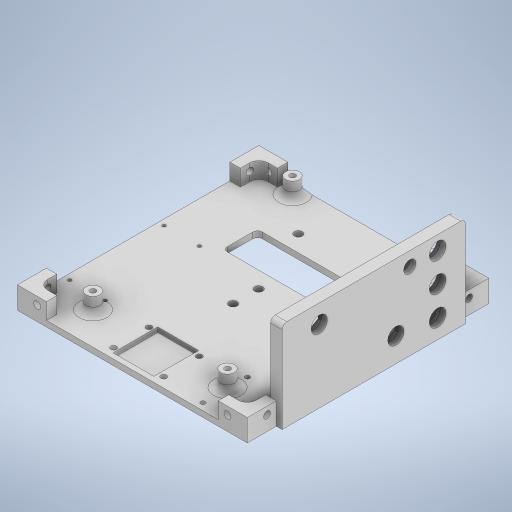
# Autodesk Inventor part: TA07 ELECTRONICS MOUNT REV 3
Saved by Autodesk Inventor 2024 (Build 280153000, 153)
## iProperties
Created: 2023-06-26
Part Number: TA07 ELECTRONICS MOUNT REV 3
Material: Generic
Document SubType Name: Modeling
Designer: TEST BENCH
Density: 1 g/cm^3
Appearance: Default
Author: TEST BENCH
Autodesk Inventor part; units mm, degrees
note: some values were not read from the file. Chosen so that the rebuilt part matches the saved one: direction of "Hole6"; direction of "Hole7".
ref_plane "YZ Plane" through (0, 0, 0) normal (1, 0, 0) x (0, 1, 0)
sketch "Sketch1" plane through (0, 0, 0) normal (0, 1, 0) x (-1, 0, 0)
  line L0 (0, 0) -> (99, 0)
  line L1 (99, 0) -> (99, -104)
  line L2 (99, -104) -> (0, -104)
  line L3 (0, -104) -> (0, 0)
  line L4 (61.8, -4.22) -> (40.2, -4.22) construction
  line L5 (40.2, -4.22) -> (40.2, -19.47) construction
  line L6 (40.2, -19.47) -> (61.8, -19.47) construction
  line L7 (61.8, -19.47) -> (61.8, -4.22) construction
  line L8 (52.5, -46.37) -> (52.5, -57.37) construction
  line L9 (64.5, -86.5) -> (37.5, -86.5) construction
  line L10 (65.8, 0) -> (36.2, 0)
  line L11 (36.2, 0) -> (36.2, -0.22)
  line L12 (36.2, -0.22) -> (65.8, -0.22)
  line L13 (65.8, -0.22) -> (65.8, 0)
  point P0 (51, -4.22)
  point P1 (36.2, 0)
  dimension "d0" = 104
  dimension "d1" = 99
  dimension "d2" = 11
  dimension "d3" = 27
  dimension "d5" = 15.25
  dimension "d6" = 21.6
  dimension "d8" = 26.9
  dimension "d11" = 17.5
  dimension "d12" = 4
  dimension "d13" = 4
  dimension "d14" = 4
  dimension "d147" = 29.13
  dimension "d202" = 2.7
  dimension "d203" = 61.5
  dimension "d204" = 46.5
  constraints: 28 end point, 8 parallel, 4 coincident, 3 horizontal, 3 perpendicular, 1 midpoint, 1 point on line
  measures "d0" distance of L0.end L1.end
  measures "d1" distance of L1.end L2.end
  measures "d2" distance of L8.end L8.start
  measures "d3" distance of L9.end L9.start
  measures "d5" distance of L6.end L4.start
  measures "d6" distance of L4.start L4.end
  measures "d8" vertical distance of L8.start L6.end
  measures "d11" distance from line of L2 L9.start
  measures "d12" distance between parallel lines of L13 L7
  measures "d13" distance from line of L12 point (51, -4.22)
  measures "d14" distance between parallel lines of L5 L11
  measures "d147" vertical distance of L9.end L8.end
  measures "d202" horizontal distance of L5.end L9.end
  measures "d203" horizontal distance of L1.end L9.end
  measures "d204" distance from line of L1 L8.end
extrude "Extrusion1" add sketch "Sketch1" against normal blind 2.5
hole "Hole1" at (-61.8, 0, -19.47) at (-61.8, 0, -4.22) at (-40.2, 0, -4.22) at (-40.2, 0, -19.47) direction (0, -1, 0) diameter 2.5 end through all
hole "Hole2" at (-52.5, 0, -46.37) at (-52.5, 0, -57.37) at (-64.5, 0, -86.5) at (-37.5, 0, -86.5) direction (0, -1, 0) diameter 3.5 end through all
sketch "Sketch2" plane through (0, -2.5, 0) normal (0, -1, 0) x (1, 0, 0)
  line L0 (-81.26, -20) -> (-96.5, -20) construction
  line L1 (-96.5, -20) -> (-96.5, -60.64) construction
  line L2 (-96.5, -60.64) -> (-81.26, -60.64) construction
  line L3 (-81.26, -60.64) -> (-81.26, -20) construction
  line L4 (-3, -36) -> (-22, -36) construction
  line L5 (-22, -36) -> (-22, -92) construction
  line L6 (-22, -92) -> (-3, -92) construction
  line L7 (-3, -92) -> (-3, -36) construction
  line L8 (-22.035, -3) -> (-22.035, -22.05) construction
  line L9 (0, -104) -> (0, 0) construction
  line L10 (-99, -104) -> (0, -104) projected
  line L11 (-12.035, -6) -> (-24.035, -6)
  line L12 (-24.035, -6) -> (-24.035, -19.05)
  line L13 (-24.035, -19.05) -> (-12.035, -19.05)
  line L14 (-12.035, -19.05) -> (-12.035, -6)
  line L15 (-0.525, -0.525) -> (-8.525, -0.525)
  line L16 (-8.525, -0.525) -> (-8.525, -24.525)
  line L17 (-8.525, -24.525) -> (-0.525, -24.525)
  line L18 (-0.525, -24.525) -> (-0.525, -0.525)
  line L19 (-0.9653, -37.5) -> (-7.5262, -37.5)
  line L20 (-7.5262, -37.5) -> (-7.5262, -51.2095)
  line L21 (-7.5262, -51.2095) -> (-0.9653, -51.2095)
  line L22 (-0.9653, -51.2095) -> (-0.9653, -37.5)
  line L23 (-13.4891, -37.5) -> (-25, -37.5)
  line L24 (-25, -37.5) -> (-25, -90.5)
  line L25 (-25, -90.5) -> (-13.4891, -90.5)
  line L26 (-13.4891, -90.5) -> (-13.4891, -37.5)
  line L27 (-79.76, -21.5) -> (-98, -21.5)
  line L28 (-98, -21.5) -> (-98, -59.14)
  line L29 (-98, -59.14) -> (-79.76, -59.14)
  line L30 (-79.76, -59.14) -> (-79.76, -21.5)
  circle A0 centre (-52.5, -57.37) radius 1.75 construction
  circle A1 centre (-64.5, -86.5) radius 1.75 construction
  line L31 (-25, -64.435) -> (-75, -64.435)
  line L32 (-75, -64.435) -> (-75, -79.435)
  line L33 (-75, -79.435) -> (-25, -79.435)
  line L34 (-25, -79.435) -> (-25, -64.435)
  line L35 (-99, 0) -> (-99, -104) projected
  line L36 (-82.7648, -21.5) -> (-94.7648, -21.5)
  line L37 (-94.7648, -21.5) -> (-94.7648, -6)
  line L38 (-94.7648, -6) -> (-82.7648, -6)
  line L39 (-82.7648, -6) -> (-82.7648, -21.5)
  line L40 (-2.5, -28.2417) -> (-10.5305, -28.2417)
  line L41 (-10.5305, -28.2417) -> (-10.5305, -31.9874)
  line L42 (-10.5305, -31.9874) -> (-2.5, -31.9874)
  line L43 (-2.5, -31.9874) -> (-2.5, -28.2417)
  line L44 (-0.191, -24.844) -> (-24.829, -24.844) construction
  line L45 (-24.829, -24.844) -> (-24.829, -0.206) construction
  line L46 (-24.829, -0.206) -> (-0.191, -0.206) construction
  line L47 (-0.191, -0.206) -> (-0.191, -24.844) construction
  line L48 (0, 0) -> (-99, 0) construction
  point P0 (-96.5, -60.64)
  point P1 (-24.035, -12.525)
  point P2 (-4.525, -24.525)
  point P3 (-4.525, -0.525)
  point P4 (-19.2445, -90.5)
  point P5 (-88.88, -20)
  point P6 (-8.525, -12.525)
  point P7 (-0.525, -12.525)
  point P8 (-25, -79.435)
  point P9 (-88.88, -21.5)
  point P10 (-75, -71.935)
  point P11 (-2.5, -30.1145)
  dimension "d32" = 19.05
  dimension "d33" = 19
  dimension "d34" = 56
  dimension "d35" = 3
  dimension "d36" = 12
  dimension "d39" = 40.64
  dimension "d40" = 15.24
  dimension "d42" = 3
  dimension "d43" = 3
  dimension "d44" = 12
  dimension "d46" = 24
  dimension "d47" = 2.475
  dimension "d48" = 1.5
  dimension "d49" = 1.5
  dimension "d50" = 1.5
  dimension "d51" = 1.5
  dimension "d52" = 1.5
  dimension "d53" = 1.5
  dimension "d56" = 15
  dimension "d58" = 50
  dimension "d59" = 8
  dimension "d148" = 1
  dimension "d189" = 29.13
  dimension "d190" = 14.565
  dimension "d191" = 25
  dimension "d192" = 12
  dimension "d193" = 15.5
  dimension "d196" = 2.5
  dimension "d221" = 24.638
  dimension "d222" = 24.638
  dimension "d223" = 2.794
  dimension "d224" = 3
  dimension "d226" = 0.334
  dimension "d227" = 0.794
  dimension "d229" = 2.794
  dimension "d230" = 0.525
  dimension "d231" = 0.525
  constraints: 90 end point, 22 parallel, 11 horizontal, 11 perpendicular, 10 coincident, 10 midpoint, 2 point on line, 1 collinear, 1 vertical
  measures "d32" distance of L8.start L8.end
  measures "d33" distance of L5.end L6.end
  measures "d34" distance of L6.end L4.start
  measures "d35" distance between parallel lines of L9 L7
  measures "d36" distance between parallel lines of L10 L6
  measures "d39" distance of L2.end L0.start
  measures "d40" distance of L0.start L0.end
  measures "d42" distance from line of L8.start L11
  measures "d43" distance from line of L8.end L13
  measures "d44" distance from line of point (-24.035, -12.525) L14
  measures "d46" distance of point (-4.525, -24.525) point (-4.525, -0.525)
  measures "d47" distance from line of L15 point (-22.035, -3)
  measures "d48" distance from line of L4.end L23
  measures "d49" vertical distance of L5.end point (-19.245, -90.5)
  measures "d50" distance from line of L0.start L27
  measures "d51" distance from line of L2.end L29
  measures "d52" distance from line of point (-96.5, -60.64) L28
  measures "d53" distance between parallel lines of L3 L30
  measures "d56" distance between parallel lines of L33 L31
  measures "d58" distance between parallel lines of L32 L34
  measures "d59" distance of point (-8.525, -12.525) point (-0.525, -12.525)
  measures "d148" distance between parallel lines of L35 L28
  measures "d189" vertical distance of A0.centre A1.centre
  measures "d190" vertical distance of A1.centre point (-75, -71.935)
  measures "d191" distance between parallel lines of L9 L24
  measures "d192" distance between parallel lines of L37 L39
  measures "d193" distance between parallel lines of L27 L38
  measures "d196" distance from line of L9 point (-2.5, -30.115)
  measures "d221" distance of L46.end L44.start
  measures "d222" distance between parallel lines of L45 L47
  measures "d223" distance from line of L46 point (-22.035, -3)
  measures "d224" distance from line of L48 point (-22.035, -3)
  measures "d226" distance between parallel lines of L47 L18
  measures "d227" distance between parallel lines of L45 L12
  measures "d229" distance between parallel lines of L45 L8
  measures "d230" distance between parallel lines of L48 L15
  measures "d231" distance between parallel lines of L9 L18
extrude "Extrusion2" cut sketch "Sketch2" against normal through all
hole "Hole3" at (-81.26, -2.5, -20) at (-81.26, -2.5, -60.64) at (-96.5, -2.5, -60.64) at (-96.5, -2.5, -20) direction (0, 1, 0) diameter 1.5 end through all
hole "Hole4" at (-22.035, -2.5, -22.05) at (-22.035, -2.5, -3) direction (0, 1, 0) diameter 2 end through all
hole "Hole5" at (-3, -2.5, -36) at (-22, -2.5, -36) at (-3, -2.5, -92) at (-22, -2.5, -92) direction (0, 1, 0) diameter 2.5 end through all
sketch "Sketch3" plane through (0, 0, 0) normal (0, 1, 0) x (1, 0, 0)
  line L0 (-60.05, 2.22) -> (-42.45, 2.22)
  line L1 (-42.45, 2.22) -> (-42.45, 21.47)
  line L2 (-42.45, 21.47) -> (-60.05, 21.47)
  line L3 (-60.05, 21.47) -> (-60.05, 2.22)
  circle A0 centre (-61.8, 4.22) radius 1.25 projected
  circle A1 centre (-40.2, 4.22) radius 1.25 projected
  circle A2 centre (-40.2, 19.47) radius 1.25 projected
  point P0 (0, 0)
  dimension "d83" = 3
  dimension "d84" = 2
  dimension "d86" = 1
  dimension "d146" = 2
  constraints: 8 end point, 2 parallel, 1 horizontal, 1 perpendicular
  measures "d84" distance from line of A1.centre L0
  measures "d86" distance edge to line of A2 L1
  measures "d146" distance from line of A2.centre L2
extrude "Extrusion3" cut sketch "Sketch3" against normal through all contours L3 L2 L1 L0
sketch "Sketch4" plane through (0, 0, 0) normal (0, 1, 0) x (1, 0, 0)
  line L0 (-80.5, 14) -> (-22.5, 14) construction
  line L1 (-22.5, 14) -> (-22.5, 100) construction
  line L2 (-22.5, 100) -> (-80.5, 100) construction
  line L3 (-80.5, 100) -> (-80.5, 14) construction
  circle A0 centre (-80.5, 14) radius 3
  circle A1 centre (-80.5, 14) radius 1.25
  circle A2 centre (-80.5, 100) radius 3
  circle A3 centre (-80.5, 100) radius 1.25
  circle A4 centre (-22.5, 100) radius 3
  circle A5 centre (-22.5, 100) radius 1.25
  circle A6 centre (-22.5, 14) radius 3
  circle A7 centre (-22.5, 14) radius 1.25
  line L4 (-99, 0) -> (0, 0) projected
  line L5 (-99, 104) -> (-99, 0) projected
  line L6 (0, 104) -> (-99, 104) projected
  point P0 (-65.136, 0)
  point P1 (-64.63, 0)
  dimension "d90" = 18.5
  dimension "d91" = 86
  dimension "d92" = 58
  dimension "d93" = 2.5
  dimension "d94" = 2.5
  dimension "d95" = 2.5
  dimension "d96" = 2.5
  dimension "d97" = 6
  dimension "d98" = 6
  dimension "d99" = 6
  dimension "d100" = 6
  dimension "d167" = 4
  constraints: 8 centre point, 8 coincident, 8 end point, 2 parallel, 1 horizontal, 1 perpendicular
  measures "d90" distance from line of L5 L0.start
  measures "d91" distance of L2.end L0.start
  measures "d92" distance of L0.start L0.end
  measures "d93" diameter of A1
  measures "d94" diameter of A3
  measures "d95" diameter of A5
  measures "d96" diameter of A7
  measures "d97" diameter of A0
  measures "d98" diameter of A2
  measures "d99" diameter of A4
  measures "d100" diameter of A6
  measures "d167" distance from line of A2.centre L6
extrude "Extrusion4" add sketch "Sketch4" along normal blind 7
sketch "Sketch5" plane through (0, 0, 0) normal (0, 1, 0) x (1, 0, 0)
  line L0 (-99, 104) -> (-99, 0) projected
  line L1 (0, 0) -> (0, 104) projected
  line L2 (-99, 0) -> (0, 0)
  line L3 (0, 0) -> (0, 104)
  line L4 (0, 104) -> (-99, 104)
  line L5 (-99, 104) -> (-99, 0)
  circle A0 centre (-96.5, 20) radius 0.75 projected
  circle A1 centre (-81.26, 20) radius 0.75 projected
  circle A2 centre (-61.8, 19.47) radius 1.25 projected
  circle A3 centre (-40.2, 19.47) radius 1.25 projected
  circle A4 centre (-96.5, 60.64) radius 0.75 projected
  circle A5 centre (-81.26, 60.64) radius 0.75 projected
  circle A6 centre (-64.5, 86.5) radius 1.75 projected
  circle A7 centre (-52.5, 57.37) radius 1.75 projected
  circle A8 centre (-52.5, 46.37) radius 1.75 projected
  circle A9 centre (-22, 36) radius 1.25 projected
  circle A10 centre (-37.5, 86.5) radius 1.75 projected
  circle A11 centre (-3, 92) radius 1.25 projected
  circle A12 centre (-22, 92) radius 1.25 projected
  circle A13 centre (-3, 36) radius 1.25 projected
  circle A14 centre (-22.035, 22.05) radius 1 projected
  circle A15 centre (-22.035, 3) radius 1 projected
  line L6 (-25, 64.435) -> (-75, 64.435) projected
  line L7 (-75, 79.435) -> (-25, 79.435) projected
  line L8 (-75, 64.435) -> (-25, 64.435)
  line L9 (-25, 64.435) -> (-25, 79.435)
  line L10 (-25, 79.435) -> (-75, 79.435)
  line L11 (-75, 79.435) -> (-75, 64.435)
  line L12 (-60.05, 2.22) -> (-60.05, 21.47) projected
  line L13 (-60.05, 21.47) -> (-42.45, 21.47) projected
  line L14 (-42.45, 21.47) -> (-42.45, 2.22) projected
  line L15 (-42.45, 2.22) -> (-60.05, 2.22) projected
  circle A16 centre (-40.2, 4.22) radius 1.25 projected
  circle A17 centre (-61.8, 4.22) radius 1.25 projected
  line L16 (-10.5305, 28.2417) -> (-10.5305, 31.9874) projected
  line L17 (-10.5305, 31.9874) -> (-2.5, 31.9874) projected
  line L18 (-2.5, 31.9874) -> (-2.5, 28.2417) projected
  line L19 (-2.5, 28.2417) -> (-10.5305, 28.2417) projected
  point P0 (-21.4439, 95.8805)
  point P1 (-23.0175, 96.2739)
  point P2 (-99, 104)
  point P3 (-58.88, 0)
  point P4 (-41.28, 0)
  point P5 (-40.23, 0)
  point P6 (-37.83, 0)
  point P7 (-22.7373, 93.0094)
  point P8 (-21.5339, 93.1598)
  point P9 (-58.88, 17.5)
  point P10 (-49.5, 2.35)
  constraints: 16 end point, 4 parallel, 2 horizontal, 2 perpendicular, 3 other
extrude "Extrusion5" add sketch "Sketch5" against normal blind 0.75
fillet "Fillet2" radius 2 6 edges at (-75, -1.25, -64.435) (-25, -0.375, -64.435) (-25, -1.625, -64.435) (-75, -1.25, -79.435) (-25, -1.625, -79.435) (-25, -0.375, -79.435)
sketch "Sketch6" plane through (0, -2.5, 0) normal (0, -1, 0) x (1, 0, 0)
  line L0 (-42.45, -2.22) -> (-42.45, -21.47) projected
  line L1 (-42.45, -21.47) -> (-60.05, -21.47) projected
  line L2 (-60.05, -21.47) -> (-60.05, -2.22) projected
  line L3 (-60.05, -2.22) -> (-42.45, -2.22) projected
  point P0 (0, 0)
  point P1 (-58.88, -17.5)
  point P2 (-49.5, -2.35)
  constraints: 2 other
extrude "Extrusion6" add sketch "Sketch6" against normal blind 0.5
ref_plane "Work Plane1" through (-49.5, 0, 0) normal (1, 0, 0) x (0, 0, -1)
sketch "Sketch7" plane through (0, 0, 0) normal (0, 1, 0) x (1, 0, 0)
  line L0 (0, 0) -> (-99, 0) projected
  line L1 (0, 0) -> (-12.5, 0)
  line L2 (-12.5, 0) -> (-12.5, 12.5)
  line L3 (-12.5, 12.5) -> (0, 12.5)
  line L4 (0, 12.5) -> (0, 0)
  line L5 (-99, 104) -> (0, 104) projected
  line L6 (0, 104) -> (-12.5, 104)
  line L7 (-12.5, 104) -> (-12.5, 91.5)
  line L8 (-12.5, 91.5) -> (0, 91.5)
  line L9 (0, 91.5) -> (0, 104)
  point P0 (-34.524, 0)
  point P1 (-6.25, 0)
  point P2 (-35.03, 0)
  point P3 (-49.5, 0)
  dimension "d111" = 12.5
  dimension "d112" = 12.5
  dimension "d113" = 12.5
  dimension "d114" = 12.5
  constraints: 16 end point, 4 parallel, 2 horizontal, 2 perpendicular, 1 midpoint
  measures "d111" distance from line of point (-6.25, 0) L3
  measures "d112" distance between parallel lines of L4 L2
  measures "d113" distance of L6.end L7.end
  measures "d114" distance of L7.end L8.end
extrude "Extrusion7" add sketch "Sketch7" along normal up to surface (7 mm away)
ref_plane "Work Plane3" through (-34.524, -2.5, 0) normal (0, 0, 1) x (1, 0, 0)
sketch "Sketch8" plane through (-34.524, -2.5, 0) normal (0, 0, 1) x (1, 0, 0)
  line L0 (34.524, 0) -> (0, 0) projected
  line L1 (34.524, 9.5) -> (22.024, 9.5) projected
  line L2 (22.024, 2.5) -> (22.024, 9.5) projected
  point P0 (34.524, 2.5)
  point P1 (26.024, 6.25)
  dimension "d117" = 9.5
  dimension "d118" = 3.25
  dimension "d119" = 4
  measures "d117" distance between parallel lines of L0 L1
  measures "d118" distance from line of L1 point (26.024, 6.25)
  measures "d119" distance from line of L2 point (26.024, 6.25)
sketch "Sketch9" plane through (0, -2.5, 0) normal (1, 0, 0) x (0, 0, -1)
  line L0 (104, 9.5) -> (91.5, 9.5) projected
  line L1 (12.5, 9.5) -> (0, 9.5) projected
  line L2 (12.5, 2.5) -> (12.5, 9.5) projected
  line L3 (91.5, 2.5) -> (91.5, 9.5) projected
  point P0 (0, 2.5)
  point P1 (8.5, 6.25)
  point P2 (95.5, 6.25)
  point P3 (91.5, 6)
  dimension "d120" = 3.25
  dimension "d121" = 3.25
  dimension "d122" = 4
  dimension "d123" = 4
  constraints: 1 midpoint
  measures "d120" distance from line of L0 point (95.5, 6.25)
  measures "d121" distance from line of L1 point (8.5, 6.25)
  measures "d122" distance from line of L2 point (8.5, 6.25)
  measures "d123" horizontal distance of point (91.5, 6) point (95.5, 6.25)
ref_plane "Work Plane2" through (-34.524, -2.5, -52) normal (0, 0, 1) x (1, 0, 0)
hole "Hole6" at (-8.5, 3.75, 0) direction (0, 0, -1) diameter 3 depth 12.5
hole "Hole7" at (0, 3.75, -8.5) at (0, 3.75, -95.5) direction (-1, 0, 0) diameter 3 depth 12.5
sketch "Sketch10" plane through (-12.5, 7, -12.5) normal (0, 1, 0) x (1, 0, 0)
  line L0 (0, 0) -> (12.5, 0) projected
  line L1 (0, 0) -> (8, 0)
  line L2 (8, 0) -> (8, -4)
  line L3 (4, -8) -> (0, -8)
  line L4 (0, -8) -> (0, 0)
  line L5 (12.5, 79) -> (0, 79) projected
  line L6 (0, 79) -> (8, 79)
  line L7 (8, 79) -> (8, 83)
  line L8 (4, 87) -> (0, 87)
  line L9 (0, 87) -> (0, 79)
  arc A0 (4, -8) -> (8, -4) centre (4, -4) ccw
  arc A1 (8, 83) -> (4, 87) centre (4, 83) ccw
  point P0 (12.5, -12.5)
  point P1 (3.1708, 0)
  point P2 (8, -8)
  point P3 (3.1708, 75)
  point P4 (8, 87)
  dimension "d138" = 8
  dimension "d139" = 8
  dimension "d140" = 8
  dimension "d141" = 8
  dimension "d142" = 4
  constraints: 16 end point, 4 parallel, 4 point on circle, 4 point on line, 4 tangent, 2 centre point, 2 horizontal, 2 perpendicular, 1 equal radius, 1 other
  measures "d138" distance of L3.end L0.start
  measures "d139" distance of point (8, -8) L3.end
  measures "d140" distance of point (8, 87) L8.end
  measures "d141" distance of L6.end point (8, 87)
  measures "d142" radius of A0
extrude "Extrusion8" cut sketch "Sketch10" against normal up to surface (7 mm away)
mirror "Mirror2" about plane through (-49.5, 0, 0) normal (1, 0, 0) of "Hole6", "Hole7", "Extrusion8", "Extrusion7"
sketch "Sketch11" plane through (0, -2.5, 0) normal (1, 0, 0) x (0, 0, -1)
  line L0 (12.5, 0) -> (91.5, 0)
  line L1 (91.5, 0) -> (91.5, 37.26)
  line L2 (89.5, 39.26) -> (14.5, 39.26)
  line L3 (12.5, 37.26) -> (12.5, 0)
  arc A0 (14.5, 39.26) -> (12.5, 37.26) centre (14.5, 37.26) ccw
  arc A1 (91.5, 37.26) -> (89.5, 39.26) centre (89.5, 37.26) ccw
  line L4 (33, 33.8581) -> (33, 28.6619)
  line L5 (33, 28.6619) -> (28.5, 26.0638)
  line L6 (28.5, 26.0638) -> (24, 28.6619)
  line L7 (24, 28.6619) -> (24, 33.8581)
  line L8 (24, 33.8581) -> (28.5, 36.4562)
  line L9 (28.5, 36.4562) -> (33, 33.8581)
  circle A2 centre (28.5, 31.26) radius 3.5
  line L10 (61.5, 15.6962) -> (66, 13.0981)
  line L11 (66, 13.0981) -> (66, 7.9019)
  line L12 (66, 7.9019) -> (61.5, 5.3038)
  line L13 (61.5, 5.3038) -> (57, 7.9019)
  line L14 (57, 7.9019) -> (57, 13.0981)
  line L15 (57, 13.0981) -> (61.5, 15.6962)
  circle A3 centre (61.5, 10.5) radius 3.5
  line L16 (12.5, 2.5) -> (12.5, 9.5) projected
  line L17 (104, 0) -> (0, 0) projected
  line L18 (91.5, 2.5) -> (91.5, 9.5) projected
  line L19 (12.5, 2.5) -> (91.5, 2.5)
  line L20 (79.5, 33.26) -> (79.5, 8.26) construction
  circle A4 centre (79.5, 33.26) radius 3.6
  circle A5 centre (79.5, 20.76) radius 3.6
  circle A6 centre (79.5, 8.26) radius 3.6
  circle A7 centre (67.5, 33.26) radius 2.65
  circle A8 centre (79.5, 33.26) radius 5
  circle A9 centre (79.5, 20.76) radius 5
  circle A10 centre (79.5, 8.26) radius 5
  circle A11 centre (67.5, 33.26) radius 4
  point P0 (91.5, -6.1595)
  point P1 (33, 55.9816)
  point P2 (24, 31.26)
  point P3 (52, 0)
  point P4 (52, 39.26)
  point P5 (91.5, 6)
  dimension "d153" = 2
  dimension "d164" = 7
  dimension "d166" = 39.26
  dimension "d171" = 9
  dimension "d173" = 9
  dimension "d174" = 7
  dimension "d177" = 24
  dimension "d182" = 0
  dimension "d184" = 0
  dimension "d185" = 0
  dimension "d188" = 2.5
  dimension "d197" = 25
  dimension "d198" = 7.2
  dimension "d199" = 7.2
  dimension "d200" = 6
  dimension "d206" = 7.2
  dimension "d207" = 5.3
  dimension "d209" = 10
  dimension "d210" = 10
  dimension "d211" = 10
  dimension "d212" = 0
  dimension "d214" = 8
  dimension "d215" = 12
  dimension "d216" = 16
  dimension "d217" = 12
  dimension "d218" = 8
  dimension "d219" = 8
  constraints: 36 end point, 12 centre point, 12 coincident, 5 midpoint, 4 parallel, 4 point on circle, 4 point on line, 4 tangent, 2 perpendicular, 1 equal radius, 26 other
  measures "d153" radius of A0
  measures "d164" diameter of A2
  measures "d166" distance from line of L0 point (52, 39.26)
  measures "d171" distance between parallel lines of L4 L7
  measures "d173" distance between parallel lines of L11 L14
  measures "d174" diameter of A3
  measures "d177" distance between parallel lines of L14 L4
  measures "d182" distance between parallel lines of L16 L3
  measures "d184" distance between parallel lines of L17 L0
  measures "d185" distance from line of point (91.5, 6) L1
  measures "d188" distance between parallel lines of L0 L19
  measures "d197" distance of L20.start L20.end
  measures "d198" diameter of A4
  measures "d199" diameter of A5
  measures "d200" distance from line of L2 point (79.5, 33.26)
  measures "d206" diameter of A6
  measures "d207" diameter of A7
  measures "d209" diameter of A8
  measures "d210" diameter of A9
  measures "d211" diameter of A10
  measures "d212" vertical distance of L20.start A7.centre
  measures "d214" diameter of A11
  measures "d215" distance from line of L1 L20.start
  measures "d216" distance from line of L3 point (28.5, 31.26)
  measures "d217" distance of L20.start A7.centre
  measures "d218" distance from line of L2 point (28.5, 31.26)
  measures "d219" distance from line of L19 A3.centre
extrude "Extrusion9" add sketch "Sketch11" along normal blind 2.5 contours L3 L19 L1 L0 | L3 A0 L2 A1 L1 L19 | L4 L5 L6 L7 L8 L9 | L10 L11 L12 L13 L14 L15 | A8 | A9 | A10 | A11
extrude "Extrusion10" add sketch "Sketch11" against normal blind 2.5 contours L3 A0 L2 A1 L1 L19
fillet "Fillet4" radius 3 4 edges at (-25.5, 0, -14) (-83.5, 0, -100) (-25.5, 0, -100) (-83.5, 0, -14)
sketch "Sketch12" plane through (0, -2.5, -104) normal (0, 0, -1) x (-1, 0, 0)
  spline S0 degree 7 poles (8.5, 7.75) (8.3869, 7.75) (8.2745, 7.7401) (8.1641, 7.7204) (8.057, 7.6915) (7.9546, 7.6541) (7.858, 7.6096) (7.727, 7.5364) (7.6874, 7.5123) (7.6491, 7.487) (7.612, 7.4606) (7.5762, 7.4332) (7.5416, 7.4048) (7.4831, 7.3532) (7.4585, 7.3304) (7.4347, 7.307) (7.4116, 7.2833) (7.3893, 7.259) (7.3677, 7.2344) (7.2618, 7.1071) (7.189, 6.9981) (7.1285, 6.8839) (7.0801, 6.7657) (7.0438, 6.6446) (7.0195, 6.5215) (7.0051, 6.3753) (7.0033, 6.3532) (7.0019, 6.3311) (7.0008, 6.309) (7.0002, 6.2868) (6.9999, 6.2647) (7.0001, 6.2232) (7.0005, 6.2039) (7.0012, 6.1846) (7.0021, 6.1653) (7.0034, 6.146) (7.0049, 6.1268) (7.0217, 5.9515) (7.0556, 5.7971) (7.1084, 5.6463) (7.1803, 5.5007) (7.2715, 5.3625) (7.3824, 5.2346) (7.5459, 5.0917) (7.5803, 5.0637) (7.6159, 5.0366) (7.6527, 5.0105) (7.6908, 4.9856) (7.7302, 4.9618) (7.8605, 4.8892) (7.9569, 4.845) (8.0589, 4.808) (8.1655, 4.7794) (8.2755, 4.7599) (8.3874, 4.75) (8.5, 4.75) knots 0 0 0 0 0 0 0 0 0.144907 0.144907 0.144907 0.144907 0.144907 0.144907 0.210638 0.210638 0.210638 0.210638 0.210638 0.210638 0.260719 0.260719 0.260719 0.260719 0.260719 0.260719 0.465238 0.465238 0.465238 0.465238 0.465238 0.465238 0.501614 0.501614 0.501614 0.501614 0.501614 0.501614 0.533311 0.533311 0.533311 0.533311 0.533311 0.533311 0.790447 0.790447 0.790447 0.790447 0.790447 0.790447 0.85561 0.85561 0.85561 0.85561 0.85561 0.85561 1 1 1 1 1 1 1 1 projected
  arc A0 (8.5, 4.75) -> (8.5, 7.75) centre (8.5, 6.25) ccw projected
  circle A1 centre (8.5, 6.25) radius 1.5 projected
  spline S1 degree 7 poles (90.5, 4.75) (90.6126, 4.75) (90.7245, 4.7599) (90.8345, 4.7794) (90.9411, 4.808) (91.0431, 4.845) (91.1395, 4.8892) (91.2698, 4.9618) (91.3092, 4.9856) (91.3473, 5.0105) (91.3841, 5.0366) (91.4197, 5.0637) (91.4541, 5.0917) (91.6176, 5.2346) (91.7285, 5.3625) (91.8197, 5.5007) (91.8916, 5.6463) (91.9444, 5.7971) (91.9783, 5.9515) (91.9951, 6.1268) (91.9966, 6.146) (91.9979, 6.1653) (91.9988, 6.1846) (91.9995, 6.2039) (91.9999, 6.2232) (92.0001, 6.2647) (91.9998, 6.2868) (91.9992, 6.309) (91.9981, 6.3311) (91.9967, 6.3532) (91.9949, 6.3753) (91.9805, 6.5215) (91.9562, 6.6446) (91.9199, 6.7657) (91.8715, 6.8839) (91.811, 6.9981) (91.7382, 7.1071) (91.6323, 7.2344) (91.6107, 7.259) (91.5884, 7.2833) (91.5653, 7.307) (91.5415, 7.3304) (91.5169, 7.3532) (91.4584, 7.4048) (91.4238, 7.4332) (91.388, 7.4606) (91.3509, 7.487) (91.3126, 7.5123) (91.273, 7.5364) (91.142, 7.6096) (91.0454, 7.6541) (90.943, 7.6915) (90.8359, 7.7204) (90.7255, 7.7401) (90.6131, 7.75) (90.5, 7.75) knots 0 0 0 0 0 0 0 0 0.14439 0.14439 0.14439 0.14439 0.14439 0.14439 0.209553 0.209553 0.209553 0.209553 0.209553 0.209553 0.466689 0.466689 0.466689 0.466689 0.466689 0.466689 0.498386 0.498386 0.498386 0.498386 0.498386 0.498386 0.534762 0.534762 0.534762 0.534762 0.534762 0.534762 0.739281 0.739281 0.739281 0.739281 0.739281 0.739281 0.789362 0.789362 0.789362 0.789362 0.789362 0.789362 0.855093 0.855093 0.855093 0.855093 0.855093 0.855093 1 1 1 1 1 1 1 1 projected
  arc A2 (90.5, 7.75) -> (90.5, 4.75) centre (90.5, 6.25) ccw projected
  circle A3 centre (90.5, 6.25) radius 1.5 projected
  constraints: 2 vertical alignment
extrude "Extrusion11" cut sketch "Sketch12" against normal up to surface (4.5 mm away)
equation "\"d13\" = d12"
equation "\"d42\" = d37"
equation "\"d43\" = d42"
equation "\"d47\" = -0.5 * d32 + 0.5 * d46"
equation "\"d51\" = d50"
equation "\"d94\" = d93"
equation "\"d95\" = d94"
equation "\"d96\" = d95"
equation "\"d98\" = d97"
equation "\"d99\" = d98"
equation "\"d100\" = d99"
equation "\"d37\" = 3"
body "Solid1"
